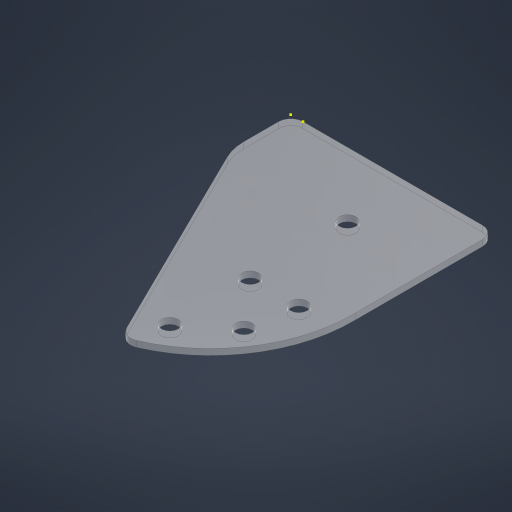
# Autodesk Inventor part: New-Sleds
Saved by Autodesk Inventor 2024 (Build 280153000, 153)
## iProperties
Created: 2023-08-23
Part Number: New-Sleds
Material: Polycarbonate, Clear
Document SubType Name: Sheet Metal
Designer: abhin
Density: 1.2 g/cm^3
Appearance: Polycarbonate - Clear
Sheet Metal Width: 2.102 in
Sheet Metal Length: 3.008 in
Sheet Metal Area: 6.324 in^2
Sheet Metal Rule: Default
Flat Pattern Width: 5.33948 cm
Flat Pattern Length: 7.64089 cm
Flat Pattern Area: 40.7984 cm^2
Author: abhin
Autodesk Inventor part; units mm, degrees
ref_plane "YZ Plane" through (0, 0, 0) normal (1, 0, 0) x (0, 1, 0)
ref_plane "XZ Plane" through (0, 0, 0) normal (0, 1, 0) x (-1, 0, 0)
ref_plane "XY Plane" through (0, 0, 0) normal (0, 0, 1) x (1, 0, 0)
sketch "Sketch9" plane through (0, 0, 0) normal (0, 1, 0) x (-1, 0, 0)
  line L0 (0, 0) -> (-53.213, 0)
  line L1 (-53.213, 0) -> (-53.213, 36.3728)
  line L2 (0, 0) -> (0, 15.24)
  line L3 (0, 15.24) -> (-28.0555, 72.2061)
  arc A0 (-28.0555, 72.2061) -> (-53.213, 36.3728) centre (-16.1162, 37.0761) ccw
  dimension "d113" = 53.213
  dimension "d114" = 36.3728
  dimension "d115" = 15.24
  dimension "d116" = 63.5
  dimension "d117" = 153.78
  constraints: 8 end point, 2 point on circle, 2 vertical, 1 centre point, 1 horizontal
  measures "d113" distance of L0.start L0.end
  measures "d114" distance of L0.end L1.end
  measures "d115" distance of L0.start L2.end
  measures "d116" distance of L2.end L3.end
  measures "d117" angle of L2 L3
extrude "Extrusion10" add sketch "Sketch9" along normal blind 1.5875
sketch "Sketch10" plane through (0, 1.5875, 0) normal (0, 1, 0) x (1, 0, 0)
  line L0 (53.213, -36.3728) -> (53.213, 0) projected
  line L1 (53.213, 0) -> (44.2468, 0)
  line L2 (53.213, 0) -> (0, 0) projected
  line L3 (44.2468, 0) -> (44.2468, -16.7386)
  line L4 (44.2468, 0) -> (44.2468, -42.1386)
  circle A0 centre (44.2468, -42.1386) radius 2.1844
  line L5 (44.2468, -42.1386) -> (31.5468, -42.1386)
  circle A1 centre (31.5468, -42.1386) radius 2.1844
  line L6 (53.213, 0) -> (27.813, 0)
  line L7 (31.5468, -42.1386) -> (31.5468, 0)
  line L8 (31.5468, -42.1386) -> (31.5468, -63.0936)
  circle A2 centre (31.5468, -63.0936) radius 2.1844
  circle A3 centre (42.0624, -54.2817) radius 2.1844
  arc A4 (31.5468, -63.0936) -> (44.2468, -42.1386) centre (25.3391, -45.0054) ccw
  line L9 (31.5468, 0) -> (31.5468, -16.7386)
  circle A5 centre (31.5468, -16.7386) radius 2.1844
  dimension "d123" = 8.9662
  dimension "d124" = 16.7386
  dimension "d126" = 42.1386
  dimension "d127" = 12.7
  dimension "d128" = 4.3688
  dimension "d129" = 25.4
  dimension "d130" = 20.955
  dimension "d131" = 4.3688
  dimension "d134" = 4.3688
  dimension "d142" = 16.7386
  dimension "d143" = 4.3688
  constraints: 16 end point, 6 centre point, 4 coincident, 4 point on line, 3 point on circle, 3 vertical, 1 horizontal, 1 perpendicular
  measures "d123" distance of L0.end L1.end
  measures "d124" distance of L1.end L3.end
  measures "d126" distance of L1.end L4.end
  measures "d127" distance of L5.start L5.end
  measures "d128" diameter of A1
  measures "d129" distance of L0.end L6.end
  measures "d130" distance of L7.start L8.end
  measures "d131" diameter of A2
  measures "d134" diameter of A3
  measures "d142" distance of L7.end L9.end
  measures "d143" diameter of A5
fillet "Fillet4" radius 3.175 2 edges at (28.0555, 0.7937, 72.2061) (53.213, 0.7937, 0)
fillet "Fillet5" radius 3.175 1 edges at (0, 0.7937, 0)
fillet "Fillet6" radius 12.7 1 edges at (0, 0.7937, 15.24)
sketch "Sketch12" plane through (0, 1.5875, 0) normal (0, 1, 0) x (1, 0, 0)
  point P0 (0, 0)
  point P1 (3.175, 0)
extrude "Extrusion13" cut sketch "Sketch10" against normal blind 1.5875 contours A5 L7 | L7 A5 | A0 A4 L4 | L4 L5 A0 | A4 A0 L5 | L7 L8 A1 | A1 L5 L7 | A1 L8 L5 | A4 A3 | A3 A4 | A2 A4 L8 | L8 A4 A2
body "Solid3"
